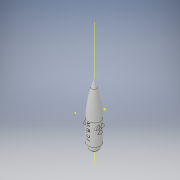
# Autodesk Inventor part: Pencil tooper
Saved by Autodesk Inventor 2018 (Build 220112000, 112)
## iProperties
Created: 2019-05-21
Part Number: Pencil tooper
Material: Generic
Document SubType Name: Modeling
Designer: 10043883
Density: 1 g/cm^3
Appearance: Default
Author: 10043883
Autodesk Inventor part; units mm, degrees
ref_plane "YZ Plane" through (0, 0, 0) normal (1, 0, 0) x (0, 1, 0)
ref_plane "XZ Plane" through (0, 0, 0) normal (0, 1, 0) x (-1, 0, 0)
ref_plane "XY Plane" through (0, 0, 0) normal (0, 0, 1) x (1, 0, 0)
sketch "Sketch1" plane through (0, 0, 0) normal (0, 0, 1) x (1, 0, 0)
  line L0 (0, 36.6275) -> (57.853, 36.6275) construction
  line L1 (25.9989, -2.9024) -> (51.3989, -2.9024)
  line L2 (25.9989, -2.9024) -> (51.3989, -2.9024)
  line L3 (51.3989, -2.9024) -> (51.3989, 38.3311)
  line L4 (51.3989, 38.3311) -> (25.9989, 38.3311)
  line L5 (25.9989, 38.3311) -> (25.9989, -2.9024)
  line L6 (38.6989, -2.9024) -> (38.6989, 38.3311)
  line L7 (25.9989, 38.3311) -> (38.6989, 82.474)
  line L8 (38.6989, 82.474) -> (51.3989, 38.3311)
  line L9 (38.6989, 82.474) -> (38.6989, 38.3311)
  line L10 (51.3989, -2.9024) -> (25.9989, -2.9024)
  line L11 (25.9989, -2.9024) -> (25.9989, -44.3081)
  line L12 (25.9989, -44.3081) -> (51.3989, -44.3081)
  line L13 (51.3989, -44.3081) -> (51.3989, -2.9024)
  line L14 (38.6989, -2.9024) -> (38.6989, -44.3081)
  point P0 (0, 0)
  point P1 (60.1022, 36.6275)
  point P2 (86.4535, -44.3081)
  dimension "d42" = 25.4
  constraints: 30 end point, 4 horizontal, 4 midpoint, 4 parallel, 3 point on line, 2 perpendicular, 1 collinear
  measures "d42" distance of L11.end L12.end
sketch "Sketch2" plane through (0, 0, 0) normal (0, 0, 1) x (1, 0, 0)
  point P0 (0, 0)
revolve "Revolution2" add sketch "Sketch1" angle 360 about axis through (38.6989, -2.9024, 0) along (0, 1, 0) contours L5 L4 L6 L1
revolve "Revolution5" add sketch "Sketch1" angle 360 about axis through (38.6989, 82.474, 0) along (0, -1, 0) contours L1 L14 L12 L11 | L7 L9 L4
hole "Hole4" at (38.6989, -44.3081, 0) direction (0, 1, 0) diameter 10.16 depth 38.1 tip angle 60
ref_plane "Work Plane9" through (38.6989, 17.7144, 12.7) normal (0, 0, -1) x (-1, 0, 0)
ref_plane "Work Plane8" through (38.6989, -44.3081, 0) normal (0, 0, -1) x (0, 1, 0)
sketch "Sketch6" plane through (38.6989, 17.7144, 12.7) normal (0, 0, -1) x (-1, 0, 0)
  line L0 (-3.4954, -41.6942) -> (-3.4954, -36.5195) construction
  line L1 (-3.4954, -36.5195) -> (31.8486, -36.5195) construction
  line L2 (31.8486, -36.5195) -> (31.8486, -41.6942) construction
  line L3 (31.8486, -41.6942) -> (-3.4954, -41.6942) construction
  line L4 (2.6638, -40.6345) -> (-3.4322, -40.6345)
  line L5 (-3.4322, -40.6345) -> (-3.4322, -40.3039)
  line L6 (-3.4322, -40.3039) -> (2.6638, -40.3039)
  line L7 (2.6638, -40.3039) -> (2.6638, -40.6345)
  line L8 (2.7805, -37.7275) -> (2.2846, -38.2525)
  line L9 (2.2846, -38.2525) -> (1.7791, -37.7275)
  line L10 (1.7791, -37.7275) -> (2.2846, -37.2073)
  line L11 (2.2846, -37.2073) -> (2.7805, -37.7275)
  line L12 (1.152, -30.7467) -> (1.8228, -31.087)
  line L13 (1.8228, -31.087) -> (2.4208, -31.7044)
  line L14 (2.4208, -31.7044) -> (2.7173, -32.3461)
  line L15 (2.7173, -32.3461) -> (2.7173, -33.5857)
  line L16 (2.7173, -33.5857) -> (2.4208, -34.2225)
  line L17 (2.4208, -34.2225) -> (1.8228, -34.8447)
  line L18 (1.8228, -34.8447) -> (1.22, -35.1413)
  line L19 (1.22, -35.1413) -> (0.345, -35.4475)
  line L20 (0.345, -35.4475) -> (-1.1085, -35.4475)
  line L21 (-1.1085, -35.4475) -> (-1.9884, -35.1413)
  line L22 (-1.9884, -35.1413) -> (-2.5912, -34.8447)
  line L23 (-2.5912, -34.8447) -> (-3.1891, -34.2225)
  line L24 (-3.1891, -34.2225) -> (-3.4954, -33.5857)
  line L25 (-3.4954, -33.5857) -> (-3.4954, -32.3461)
  line L26 (-3.4954, -32.3461) -> (-3.1891, -31.7044)
  line L27 (-3.1891, -31.7044) -> (-2.5912, -31.087)
  line L28 (-2.5912, -31.087) -> (-1.9203, -30.7467)
  line L29 (-1.9203, -30.7467) -> (-1.7599, -31.0384)
  line L30 (-1.7599, -31.0384) -> (-2.3919, -31.369)
  line L31 (-2.3919, -31.369) -> (-2.9169, -31.9086)
  line L32 (-2.9169, -31.9086) -> (-3.1697, -32.4238)
  line L33 (-3.1697, -32.4238) -> (-3.1697, -33.503)
  line L34 (-3.1697, -33.503) -> (-2.9169, -34.0232)
  line L35 (-2.9169, -34.0232) -> (-2.3919, -34.5628)
  line L36 (-2.3919, -34.5628) -> (-1.8669, -34.8399)
  line L37 (-1.8669, -34.8399) -> (-1.0647, -35.1121)
  line L38 (-1.0647, -35.1121) -> (0.2964, -35.1121)
  line L39 (0.2964, -35.1121) -> (1.0985, -34.8399)
  line L40 (1.0985, -34.8399) -> (1.6235, -34.5628)
  line L41 (1.6235, -34.5628) -> (2.1485, -34.0232)
  line L42 (2.1485, -34.0232) -> (2.4013, -33.503)
  line L43 (2.4013, -33.503) -> (2.4013, -32.4238)
  line L44 (2.4013, -32.4238) -> (2.1485, -31.9086)
  line L45 (2.1485, -31.9086) -> (1.6235, -31.369)
  line L46 (1.6235, -31.369) -> (0.9916, -31.0384)
  line L47 (0.9916, -31.0384) -> (1.152, -30.7467)
  line L48 (2.7805, -27.3244) -> (2.2846, -27.8494)
  line L49 (2.2846, -27.8494) -> (1.7791, -27.3244)
  line L50 (1.7791, -27.3244) -> (2.2846, -26.8042)
  line L51 (2.2846, -26.8042) -> (2.7805, -27.3244)
  line L52 (-0.5251, -21.4569) -> (-0.389, -21.0291)
  line L53 (-0.389, -21.0291) -> (-0.0585, -20.6839)
  line L54 (-0.0585, -20.6839) -> (0.5638, -20.368)
  line L55 (0.5638, -20.368) -> (1.4825, -20.368)
  line L56 (1.4825, -20.368) -> (2.0999, -20.6839)
  line L57 (2.0999, -20.6839) -> (2.4256, -21.0291)
  line L58 (2.4256, -21.0291) -> (2.7173, -21.9576)
  line L59 (2.7173, -21.9576) -> (2.7173, -24.7528)
  line L60 (2.7173, -24.7528) -> (-3.4954, -24.7528)
  line L61 (-3.4954, -24.7528) -> (-3.4954, -21.9576)
  line L62 (-3.4954, -21.9576) -> (-3.194, -21.0291)
  line L63 (-3.194, -21.0291) -> (-2.8731, -20.6839)
  line L64 (-2.8731, -20.6839) -> (-2.246, -20.368)
  line L65 (-2.246, -20.368) -> (-1.6092, -20.368)
  line L66 (-1.6092, -20.368) -> (-0.987, -20.6839)
  line L67 (-0.987, -20.6839) -> (-0.6613, -21.0291)
  line L68 (-0.6613, -21.0291) -> (-0.5251, -21.4569)
  line L69 (-0.3599, -22.0062) -> (-0.3599, -24.4222)
  line L70 (-0.3599, -24.4222) -> (2.4013, -24.4222)
  line L71 (2.4013, -24.4222) -> (2.4013, -22.0062)
  line L72 (2.4013, -22.0062) -> (2.1437, -21.2041)
  line L73 (2.1437, -21.2041) -> (1.9055, -20.9659)
  line L74 (1.9055, -20.9659) -> (1.3999, -20.7034)
  line L75 (1.3999, -20.7034) -> (0.6367, -20.7034)
  line L76 (0.6367, -20.7034) -> (0.136, -20.9659)
  line L77 (0.136, -20.9659) -> (-0.1022, -21.2041)
  line L78 (-0.1022, -21.2041) -> (-0.3599, -22.0062)
  line L79 (-0.6856, -24.4222) -> (-0.6856, -22.0062)
  line L80 (-0.6856, -22.0062) -> (-0.9432, -21.2041)
  line L81 (-0.9432, -21.2041) -> (-1.1863, -20.9659)
  line L82 (-1.1863, -20.9659) -> (-1.687, -20.7034)
  line L83 (-1.687, -20.7034) -> (-2.1683, -20.7034)
  line L84 (-2.1683, -20.7034) -> (-2.6738, -20.9659)
  line L85 (-2.6738, -20.9659) -> (-2.912, -21.2041)
  line L86 (-2.912, -21.2041) -> (-3.1697, -22.0062)
  line L87 (-3.1697, -22.0062) -> (-3.1697, -24.4222)
  line L88 (-3.1697, -24.4222) -> (-0.6856, -24.4222)
  line L89 (2.7805, -16.9213) -> (2.2846, -17.4463)
  line L90 (2.2846, -17.4463) -> (1.7791, -16.9213)
  line L91 (1.7791, -16.9213) -> (2.2846, -16.4012)
  line L92 (2.2846, -16.4012) -> (2.7805, -16.9213)
  line L93 (2.6638, -9.3864) -> (2.6638, -9.717)
  line L94 (2.6638, -9.717) -> (-2.4551, -9.717)
  line L95 (-2.4551, -9.717) -> (2.6638, -11.7295)
  line L96 (2.6638, -11.7295) -> (2.6638, -12.0018)
  line L97 (2.6638, -12.0018) -> (-2.4551, -14.0192)
  line L98 (-2.4551, -14.0192) -> (2.6638, -14.0192)
  line L99 (2.6638, -14.0192) -> (2.6638, -14.3497)
  line L100 (2.6638, -14.3497) -> (-3.4322, -14.3497)
  line L101 (-3.4322, -14.3497) -> (-3.4322, -14.0483)
  line L102 (-3.4322, -14.0483) -> (2.1145, -11.8656)
  line L103 (2.1145, -11.8656) -> (-3.4322, -9.6878)
  line L104 (-3.4322, -9.6878) -> (-3.4322, -9.3864)
  line L105 (-3.4322, -9.3864) -> (2.6638, -9.3864)
  point P0 (38.6989, -17.7144)
  constraints: 2 other
extrude "Extrusion3" add sketch "Sketch6" along normal blind 25.4
ref_plane "Work Plane10" through (51.3989, -2.9024, 0) normal (1, 0, 0) x (0, 1, 0)
fillet "Fillet5" radius 196.85 1 edges at (51.3989, 38.3311, 0)
sketch "Sketch7" plane through (51.3989, -2.9024, 0) normal (1, 0, 0) x (0, 1, 0)
  line L0 (0.2488, 2.5647) -> (0.2488, -2.5647) projected
  circle A0 centre (0.2488, 0) radius 10.3788
  arc A1 (8.5027, 1.9887) -> (1.1594, 9.0888) centre (-0.0471, 0.4934) ccw
  line L1 (1.1594, 9.0888) -> (0.276, 3.4875)
  line L2 (8.5027, 1.9887) -> (2.844, 1.4137)
  arc A2 (2.844, 1.4137) -> (0.276, 3.4875) centre (-0.4963, -0.0957) ccw
  circle A3 centre (0.2488, 0) radius 2.2322
  arc A4 (0.8722, -9.1023) -> (8.4313, -2.2325) centre (-0.0683, -0.4738) ccw
  line L3 (8.4313, -2.2325) -> (2.8987, -0.9894)
  line L4 (0.8722, -9.1023) -> (0.6635, -3.4182)
  arc A5 (0.6635, -3.4182) -> (2.8987, -0.9894) centre (-0.6272, 0.0125) ccw
  arc A6 (-7.9804, 4.8535) -> (-7.5597, -4.9877) centre (-0.6296, 0.2381) ccw
  line L5 (-7.5597, -4.9877) -> (-2.9749, -1.6509)
  line L6 (-7.9804, 4.8535) -> (-2.9749, 1.4137)
  arc A7 (-2.9749, 1.4137) -> (-2.9749, -1.6509) centre (0.355, -0.1186) ccw
  point P0 (2.9024, 0)
  constraints: 12 end point, 12 point on circle, 8 centre point, 1 coincident, 1 midpoint
extrude "Extrusion4" add sketch "Sketch7" against normal blind 25.4 contours A3 L0 | L0 A3 | L2 A2 L1 A1 | L4 A5 L3 A4 | L6 A7 L5 A6
chamfer "Chamfer1" distance 5.715 angle 45 1 edges at (51.3989, -44.3081, 0)
chamfer "Chamfer2" distance 5.715 angle 45 1 edges at (51.3989, -38.5931, 0)
body "Solid1"
